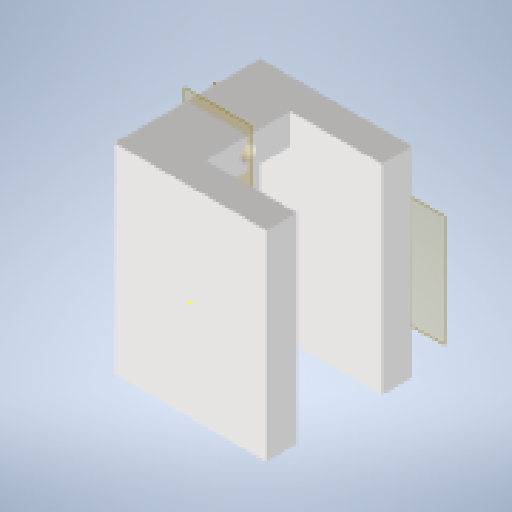
# Autodesk Inventor part: roka4
Saved by Autodesk Inventor 2023.2 (Build 272271000, 271)
## iProperties
Created: 2023-09-06
Part Number: roka4
Material: Generic
Document SubType Name: Modeling
Designer: jebes windows
Density: 1 g/cm^3
Appearance: Default
Author: jebes windows
Autodesk Inventor part; units mm, degrees
ref_plane "YZ Plane" through (0, 0, 0) normal (1, 0, 0) x (0, 1, 0)
ref_plane "XZ Plane" through (0, 0, 0) normal (0, 1, 0) x (-1, 0, 0)
ref_plane "XY Plane" through (0, 0, 0) normal (0, 0, 1) x (1, 0, 0)
ref_plane "Work Plane1" through (0, 0, 0) normal (0, 0, 1) x (1, 0, 0)
sketch "Sketch1" plane through (0, 0, 0) normal (0, 0, 1) x (1, 0, 0)
  line L0 (1.9, -6.45) -> (1.9, -2.8797) projected
  arc A0 (1.9, -2.8797) -> (2.2091, -2.65) centre (0, 0) ccw projected
  line L1 (2.2091, -2.65) -> (14.1591, -1.997) projected
  arc A1 (14.1591, -1.997) -> (14.1591, 1.997) centre (14.05, 0) ccw projected
  line L2 (14.1591, 1.997) -> (2.2091, 2.65) projected
  arc A2 (2.2091, 2.65) -> (1.9, 2.8797) centre (0, 0) ccw projected
  line L3 (1.9, 2.8797) -> (1.9, 6.45) projected
  arc A3 (1.9, 6.45) -> (-1.9, 6.45) centre (0, 6.45) ccw projected
  line L4 (-1.9, 6.45) -> (-1.9, 3.2953) projected
  line L5 (-1.9, 3.2953) -> (-16.6263, 1.9922) projected
  arc A4 (-16.6263, 1.9922) -> (-16.6263, -1.9922) centre (-16.45, 0) ccw projected
  line L6 (-16.6263, -1.9922) -> (-1.9, -3.2953) projected
  line L7 (-1.9, -3.2953) -> (-1.9, -6.45) projected
  arc A5 (-1.9, -6.45) -> (1.9, -6.45) centre (0, -6.45) ccw projected
  circle A6 centre (-14.85, 0) radius 0.6 projected
  circle A7 centre (-16.85, 0) radius 0.6 projected
  circle A8 centre (-12.85, 0) radius 0.6 projected
  circle A9 centre (-10.85, 0) radius 0.6 projected
  circle A10 centre (-8.85, 0) radius 0.6 projected
  circle A11 centre (-6.85, 0) radius 0.6 projected
  circle A12 centre (-4.85, 0) radius 0.6 projected
  circle A13 centre (4.45, 0) radius 0.6 projected
  circle A14 centre (6.45, 0) radius 0.6 projected
  circle A15 centre (8.45, 0) radius 0.6 projected
  circle A16 centre (10.45, 0) radius 0.6 projected
  circle A17 centre (14.45, 0) radius 0.6 projected
  circle A18 centre (12.45, 0) radius 0.6 projected
  circle A19 centre (0, 0) radius 2.3 projected
  circle A20 centre (0, -4.45) radius 0.6 projected
  circle A21 centre (0, -6.45) radius 0.6 projected
  circle A22 centre (0, 4.45) radius 0.6 projected
  circle A23 centre (0, 6.45) radius 0.6 projected
  line L8 (12.5, 16.5) -> (-12.5, 16.5)
  line L9 (-12.5, 16.5) -> (-12.5, -16.5)
  line L10 (-12.5, -16.5) -> (12.5, -16.5)
  line L11 (12.5, -16.5) -> (12.5, 16.5)
  line L12 (12.5, 16.5) -> (-12.5, -16.5) construction
  line L13 (-12.5, 16.5) -> (12.5, -16.5) construction
  point P0 (0, 0)
  dimension "d0" = 25
  dimension "d1" = 33
  constraints: 12 end point, 2 midpoint, 2 parallel, 1 horizontal, 1 perpendicular
  measures "d0" distance of L10.end L9.end
  measures "d1" distance of L9.end L8.end
extrude "Extrusion1" add sketch "Sketch1" along normal blind 5 contours A5 L7 L6 L9 A8 L5 L4 A3 L3 A2 L2 L11 A18 L1 A0 L0 | L0 A0 L1 L11 L10 L9 L6 L7 A5 | A18 L11 | L9 A8 | L2 A2 L3 A3 L4 L5 L9 L8 L11 | A9 | A10 | A11 | A12 | A13 | A14 | A15 | A16 | A19 | A20 | A21 | A22 | A23 picked at (12.2127, -0.0768) picked at (-12.4038, -0.1232)
sketch "Sketch2" plane through (0, 0, 5) normal (0, 0, 1) x (1, 0, 0)
  line L0 (-12.5, 16.5) -> (-12.5, -16.5) projected
  line L1 (-12.5, -16.5) -> (-7.5, -16.5)
  line L2 (-12.5, -16.5) -> (12.5, -16.5) projected
  line L3 (-7.5, -16.5) -> (-7.5, 16.5)
  line L4 (12.5, 16.5) -> (-12.5, 16.5) projected
  line L5 (-12.5, 16.5) -> (-7.5, 16.5)
  line L6 (-12.5, 16.5) -> (-12.5, -16.5)
  point P0 (0, 0)
  dimension "d4" = 5
  constraints: 8 end point, 2 collinear, 2 point on line, 1 perpendicular
  measures "d4" distance of L0.end L1.end
extrude "Extrusion2" add sketch "Sketch2" along normal blind 14
sketch "Sketch3" plane through (-7.5, -16.5, 5) normal (1, 0, 0) x (0, 0, -1)
  line L0 (0, 0) -> (0, 33) projected
  line L1 (0, 0) -> (0, 5)
  line L2 (0, 5) -> (-14, 5)
  line L3 (-14, 33) -> (-14, 0) projected
  line L4 (-14, 0) -> (-14, 5)
  line L5 (5, 0) -> (-14, 0) projected
  line L6 (-14, 0) -> (0, 0)
  line L7 (0, 33) -> (0, 28)
  line L8 (0, 28) -> (-14, 28)
  line L9 (5, 33) -> (-14, 33) projected
  line L10 (-14, 28) -> (-14, 33)
  line L11 (-14, 33) -> (0, 33)
  circle A0 centre (-7, 2.5) radius 1.25
  circle A1 centre (-7, 30.5) radius 1.25
  point P0 (5, 16.5)
  point P1 (-14, 30.5)
  dimension "d7" = 5
  dimension "d8" = 5
  dimension "d9" = 2.5
  dimension "d10" = 2.5
  dimension "d11" = 2.5
  dimension "d12" = 7
  dimension "d13" = 2.5
  dimension "d14" = 7
  constraints: 16 end point, 4 point on line, 2 centre point, 2 collinear, 2 perpendicular, 1 midpoint, 1 vertical
  measures "d7" distance of L0.start L1.end
  measures "d8" distance of L0.end L7.end
  measures "d9" diameter of A0
  measures "d10" diameter of A1
  measures "d11" distance from line of L9 A1.centre
  measures "d12" distance of point (-14, 30.5) A1.centre
  measures "d13" distance from line of L2 A0.centre
  measures "d14" distance from line of L4 A0.centre
extrude "Extrusion3" add sketch "Sketch3" along normal blind 5 contours L5 L3 L2 L0 | L8 L3 L9 L0
sketch "Sketch4" plane through (-7.5, -11.5, 5) normal (1, 0, 0) x (0, 0, -1)
  point P0 (5, 11.5)
sketch "Sketch5" plane through (-7.5, -11.5, 5) normal (1, 0, 0) x (0, 0, -1)
  circle A0 centre (-7, 6) radius 6.25
  circle A1 centre (-7, 12.25) radius 3.25
  line L0 (-14, -5) -> (0, -5) projected
  line L1 (-14, 0) -> (-14, 23) projected
  point P0 (5, 11.5)
  point P1 (-10.1382, 11.405)
  point P2 (-3.8618, 11.405)
  dimension "d17" = 12.5
  dimension "d18" = 6.5
  dimension "d19" = 11
  dimension "d20" = 7
  dimension "d21" = 7
  constraints: 1 centre point, 3 other
  measures "d18" diameter of A1
  measures "d19" distance from line of L0 point (-7, 6)
  measures "d20" distance from line of L1 point (-7, 6)
  measures "d21" distance from line of L1 A1.centre
extrude "Extrusion4" cut sketch "Sketch5" against normal blind 5
ref_plane "Work Plane2" through (0, 0, 12) normal (0, 0, 1) x (1, 0, 0)
mirror "Mirror1" about plane through (0, 0, 12) normal (0, 0, 1) of "Extrusion1"
sketch "Sketch6" plane through (-12.5, 16.5, 24) normal (0, 0, 1) x (1, 0, 0)
  line L0 (25, 0) -> (0, 0) projected
  line L1 (0, 0) -> (0, -33) projected
  line L2 (0, -33) -> (25, -33) projected
  line L3 (25, -33) -> (25, 0) projected
  point P0 (12.5, -16.5)
extrude "Extrusion5" cut sketch "Sketch6" against normal blind 2
body "Solid1"
